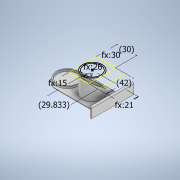
# Autodesk Inventor part: RV
Saved by Autodesk Inventor 2021 (Build 250183000, 183)
## iProperties
Created: 2020-06-05
Part Number: RV
Material: Generic
Document SubType Name: Modeling
Designer: andre
Density: 1 g/cm^3
Appearance: Default
Author: andre
## iProperties of the stored document _3DPrint.ipt
Created: 2020-06-05
Part Number: _3DPrint
Material: Generic
Document SubType Name: Modeling
Designer: andre
Density: 1 g/cm^3
Appearance: Default
Author: andre
Autodesk Inventor part; units mm, degrees
ref_plane "YZ Plane" through (0, 0, 0) normal (1, 0, 0) x (0, 1, 0)
ref_plane "XZ Plane" through (0, 0, 0) normal (0, 1, 0) x (-1, 0, 0)
ref_plane "XY Plane" through (0, 0, 0) normal (0, 0, 1) x (1, 0, 0)
sketch "Sketch1" plane through (0, 0, 0) normal (0, 1, 0) x (-1, 0, 0)
  line L0 (0, 0) -> (85, 0)
  line L1 (85, 0) -> (85, -42)
  line L2 (85, -42) -> (0, -42)
  line L3 (0, -42) -> (0, 0)
  dimension "d0" = 85
  dimension "d1" = 42
  constraints: 8 end point, 2 parallel, 1 horizontal, 1 perpendicular
  measures "d0" distance of L1.end L2.end
  measures "d1" distance of L0.end L1.end
extrude "Extrusion1" add sketch "Sketch1" along normal blind 1
sketch "Sketch2" plane through (0, 1, 0) normal (0, 1, 0) x (1, 0, 0)
  line L0 (-44.8327, 0) -> (-14.8327, 0)
  line L1 (-14.8327, 0) -> (-14.8327, 42)
  line L2 (-14.8327, 42) -> (-44.8327, 42)
  line L3 (-44.8327, 42) -> (-44.8327, 0)
  line L4 (-85, 0) -> (0, 0) projected
  dimension "d4" = 42
  dimension "d5" = 30
  dimension "d6" = 0
  constraints: 8 end point, 2 parallel, 1 horizontal, 1 perpendicular
  measures "d4" distance between parallel lines of L2 L0
  measures "d5" distance between parallel lines of L1 L3
  measures "d6" distance between parallel lines of L4 L0
extrude "Extrusion2" add sketch "Sketch2" along normal blind 32
sketch "Sketch5" plane through (0, 33, 0) normal (0, 1, 0) x (1, 0, 0)
  circle A0 centre (-29.8327, 21) radius 13
  line L0 (-44.8327, 42) -> (-44.8327, 0) projected
  line L1 (-44.8327, 0) -> (-14.8327, 0) projected
  line L2 (-14.8327, 0) -> (-14.8327, 42) projected
  line L3 (-14.8327, 42) -> (-44.8327, 42) projected
  circle A1 centre (-29.8327, 21) radius 15
  line L4 (0, 0) -> (0, 42) projected
  point P0 (-24.115, 0)
  point P1 (-44.8327, 21)
  point P2 (-14.8327, 21)
  point P3 (-19.6709, 0)
  dimension "d20" = 26
  dimension "d21" = 15
  dimension "d22" = 21
  dimension "d23" = 30
  dimension "d24" = 42
  dimension "d34" = 30
  dimension "d63" = 29.8327
  constraints: 2 centre point, 1 coincident
  measures "d20" diameter of A0
  measures "d21" distance from line of L0 A0.centre
  measures "d22" distance from line of L1 A0.centre
  measures "d23" distance between parallel lines of L2 L0
  measures "d24" distance between parallel lines of L3 L1
  measures "d34" diameter of A1
  measures "d63" distance from line of L4 A0.centre
extrude "Extrusion3" cut sketch "Sketch5" against normal blind 32 contours A0
chamfer "Chamfer3" distance 42 distance2 32 1 edges at (-29.8327, 33, -42)
extrude "Extrusion4" cut sketch "Sketch5" against normal blind 32 contours L3 L2 A1 L0 | A1 L2 L1 L0
sketch "Sketch6" plane through (0, 1, 0) normal (0, 1, 0) x (1, 0, 0)
  circle A0 centre (-68, 21) radius 15.75
  line L0 (-85, 0) -> (0, 0) projected
  circle A1 centre (-68, 21) radius 17
  line L1 (-85, 42) -> (-85, 0) projected
  point P0 (-28.5591, 0)
  dimension "d37" = 31.5
  dimension "d38" = 21
  dimension "d39" = 34
  dimension "d64" = 17
  constraints: 2 centre point, 1 coincident
  measures "d37" diameter of A0
  measures "d38" distance from line of L0 A0.centre
  measures "d39" diameter of A1
  measures "d64" distance from line of L1 A1.centre
extrude "Extrusion5" add sketch "Sketch6" along normal blind 3
fillet "Fillet3" radius 21 2 edges at (-85, 0.5, 0) (-85, 0.5, -42)
sketch "Sketch9" plane through (0, 0, 0) normal (1, 0, 0) x (0, 0, -1)
  line L0 (-11.5, 0) -> (53.5, 0)
  line L1 (53.5, 0) -> (53.5, 1)
  line L2 (53.5, 1) -> (-11.5, 1)
  line L3 (-11.5, 1) -> (-11.5, 0)
  line L4 (0, 0) -> (0, 1) projected
  dimension "d49" = 1
  dimension "d50" = 65
  dimension "d53" = 11.5
  constraints: 8 end point, 2 parallel, 1 horizontal, 1 perpendicular
  measures "d49" distance of L1.end L0.end
  measures "d50" distance between parallel lines of L1 L3
  measures "d53" distance between parallel lines of L3 L4
extrude "Extrusion8" add sketch "Sketch9" along normal blind 2
sketch "Sketch10" plane through (0, 1, 0) normal (0, 1, 0) x (1, 0, 0)
  line L0 (0, -11.5) -> (0, 0) projected
  line L1 (2, 53.5) -> (2, -11.5) projected
  line L2 (0, -11.5) -> (2, -11.5)
  line L3 (2, -11.5) -> (2, 53.5)
  line L4 (2, 53.5) -> (0, 53.5)
  line L5 (0, 53.5) -> (0, -11.5)
  point P0 (2, -11.5)
  constraints: 8 end point, 2 parallel, 1 horizontal, 1 perpendicular
extrude "Extrusion9" add sketch "Sketch10" along normal blind 15
sketch "Sketch11" plane through (0, 0, 0) normal (-1, 0, 0) x (0, 0, 1)
  line L0 (11.5, 0) -> (-53.5, 0) projected
  line L1 (-53.5, 6) -> (-42, 6)
  line L2 (-42, 6) -> (-42, 0)
  line L3 (-42, 0) -> (-53.5, 0)
  line L4 (-53.5, 0) -> (-53.5, 6)
  line L5 (-53.5, 16) -> (11.5, 16) projected
  line L6 (-53.5, 0) -> (-53.5, 16) projected
  point P0 (0, 0)
  dimension "d56" = 11.5
  dimension "d58" = 0
  dimension "d65" = 6
  constraints: 8 end point, 2 parallel, 1 horizontal, 1 perpendicular, 1 point on line
  measures "d56" distance of L2.end L3.end
  measures "d58" distance between parallel lines of L6 L4
  measures "d65" distance between parallel lines of L1 L0
extrude "Extrusion10" add sketch "Sketch11" along normal blind 6
fillet "Fillet4" radius 5.9 1 edges at (-6, 6, -47.75)
fillet "Fillet5" radius 2 1 edges at (2, 16, -21)
sketch "Sketch12" plane through (0, 1, 0) normal (0, 1, 0) x (1, 0, 0)
  line L0 (-4.5, 34) -> (-10.3327, 34)
  line L1 (-10.3327, 34) -> (-10.3327, 8)
  line L2 (-10.3327, 8) -> (-4.5, 8)
  line L3 (-4.5, 8) -> (-4.5, 34)
  line L4 (-5.931, 42) -> (-64, 42) projected
  line L5 (-64, 0) -> (0, 0) projected
  line L6 (0, 53.5) -> (0, -11.5) projected
  circle A0 centre (-29.8327, 21) radius 15 projected
  dimension "d66" = 8
  dimension "d67" = 8
  dimension "d68" = 4.5
  dimension "d69" = 4.5
  constraints: 8 end point, 2 parallel, 1 horizontal, 1 perpendicular
  measures "d66" distance between parallel lines of L4 L0
  measures "d67" distance between parallel lines of L5 L2
  measures "d68" distance between parallel lines of L6 L3
  measures "d69" distance edge to line of A0 L1
extrude "Extrusion11" add sketch "Sketch12" along normal blind 2 contours L3 L2 L1 L0
sketch "Sketch13" plane through (0, 3, 0) normal (0, 1, 0) x (1, 0, 0)
  line L0 (-4.5, 34) -> (-4.5, 8) construction
  line L1 (-4.5, 8) -> (-10.3327, 8) construction
  line L2 (-10.3327, 8) -> (-10.3327, 34) construction
  line L3 (-10.3327, 34) -> (-4.5, 34) construction
  line L4 (-4.5, 34) -> (-10.3327, 34) projected
  line L5 (-10.3327, 8) -> (-4.5, 8) projected
  line L6 (-4.5, 8) -> (-4.5, 34) projected
  line L7 (-10.3327, 34) -> (-10.3327, 8) projected
  spline S0 degree 2 poles (-8.9212, 32.0386) (-8.9188, 31.8937) (-8.7545, 31.7343) (-8.6024, 31.7319) knots 0 0 0 1 2 2 2
  line L8 (-8.6024, 31.7319) -> (-7.8101, 31.7319)
  line L9 (-7.8101, 31.7319) -> (-7.8101, 31.2126)
  line L10 (-7.8101, 31.2126) -> (-8.6893, 30.7271)
  spline S1 degree 2 poles (-8.6893, 30.7271) (-8.8197, 30.657) (-8.9236, 30.5217) (-8.9212, 30.4155) knots 0 0 0 1 2 2 2
  spline S2 degree 2 poles (-8.9212, 30.4155) (-8.9188, 30.2802) (-8.7642, 30.1111) (-8.641, 30.1063) knots 0 0 0 1 2 2 2
  spline S3 degree 2 poles (-8.641, 30.1063) (-8.5903, 30.1063) (-8.4937, 30.1353) (-8.4309, 30.1715) knots 0 0 0 1 2 2 2
  line L11 (-8.4309, 30.1715) -> (-7.7014, 30.5942)
  spline S4 degree 2 poles (-7.7014, 30.5942) (-7.5951, 30.3502) (-7.1652, 30.0918) (-6.8874, 30.0918) knots 0 0 0 1 2 2 2
  spline S5 degree 2 poles (-6.8874, 30.0918) (-6.4502, 30.0942) (-5.9623, 30.6401) (-5.9574, 31.1473) knots 0 0 0 1 2 2 2
  line L12 (-5.9574, 31.1473) -> (-5.9574, 32.0386)
  spline S6 degree 2 poles (-5.9574, 32.0386) (-5.9574, 32.1836) (-6.1241, 32.343) (-6.2738, 32.343) knots 0 0 0 1 2 2 2
  line L13 (-6.2738, 32.343) -> (-8.6024, 32.343)
  spline S7 degree 2 poles (-8.6024, 32.343) (-8.7545, 32.343) (-8.9188, 32.1836) (-8.9212, 32.0386) knots 0 0 0 1 2 2 2
  line L14 (-7.3656, 31.7319) -> (-6.4357, 31.7319)
  line L15 (-6.4357, 31.7319) -> (-6.4357, 31.2126)
  spline S8 degree 2 poles (-6.4357, 31.2126) (-6.4381, 30.9831) (-6.6845, 30.7222) (-6.8995, 30.7198) knots 0 0 0 1 2 2 2
  spline S9 degree 2 poles (-6.8995, 30.7198) (-7.1193, 30.7198) (-7.3632, 30.9734) (-7.3656, 31.2077) knots 0 0 0 1 2 2 2
  line L16 (-7.3656, 31.2077) -> (-7.3656, 31.7319)
  spline S10 degree 2 poles (-8.9164, 29.4179) (-8.9164, 29.2899) (-8.7666, 29.1473) (-8.6313, 29.1473) knots 0 0 0 1 2 2 2
  line L17 (-8.6313, 29.1473) -> (-6.9067, 29.1473)
  line L18 (-6.9067, 29.1473) -> (-6.9067, 29.1304)
  line L19 (-6.9067, 29.1304) -> (-8.6748, 28.4082)
  spline S11 degree 2 poles (-8.6748, 28.4082) (-8.769, 28.372) (-8.8608, 28.2391) (-8.8584, 28.1425) knots 0 0 0 1 2 2 2
  spline S12 degree 2 poles (-8.8584, 28.1425) (-8.8608, 28.0483) (-8.769, 27.9203) (-8.6724, 27.8816) knots 0 0 0 1 2 2 2
  line L20 (-8.6724, 27.8816) -> (-6.9067, 27.1594)
  line L21 (-6.9067, 27.1594) -> (-6.9067, 27.1425)
  line L22 (-6.9067, 27.1425) -> (-8.6313, 27.1425)
  spline S13 degree 2 poles (-8.6313, 27.1425) (-8.7666, 27.1425) (-8.9164, 27.0024) (-8.9164, 26.872) knots 0 0 0 1 2 2 2
  spline S14 degree 2 poles (-8.9164, 26.872) (-8.9164, 26.7415) (-8.7666, 26.599) (-8.6313, 26.599) knots 0 0 0 1 2 2 2
  line L23 (-8.6313, 26.599) -> (-6.3101, 26.599)
  spline S15 degree 2 poles (-6.3101, 26.599) (-6.1241, 26.6014) (-5.9188, 26.8043) (-5.9164, 26.9928) knots 0 0 0 1 2 2 2
  spline S16 degree 2 poles (-5.9164, 26.9928) (-5.9164, 27.1498) (-6.0661, 27.3502) (-6.2328, 27.4155) knots 0 0 0 1 2 2 2
  line L24 (-6.2328, 27.4155) -> (-8.0275, 28.1377)
  line L25 (-8.0275, 28.1377) -> (-8.0275, 28.1546)
  line L26 (-8.0275, 28.1546) -> (-6.2328, 28.8792)
  spline S17 degree 2 poles (-6.2328, 28.8792) (-6.0637, 28.942) (-5.9139, 29.1401) (-5.9164, 29.2971) knots 0 0 0 1 2 2 2
  spline S18 degree 2 poles (-5.9164, 29.2971) (-5.9188, 29.4855) (-6.1241, 29.6908) (-6.3101, 29.6908) knots 0 0 0 1 2 2 2
  line L27 (-6.3101, 29.6908) -> (-8.6313, 29.6908)
  spline S19 degree 2 poles (-8.6313, 29.6908) (-8.7666, 29.6908) (-8.9164, 29.5483) (-8.9164, 29.4179) knots 0 0 0 1 2 2 2
  line L28 (-8.8777, 24.9903) -> (-8.8777, 24.0024)
  spline S20 degree 2 poles (-8.8777, 24.0024) (-8.8729, 23.529) (-8.4309, 22.9976) (-8.042, 22.9928) knots 0 0 0 1 2 2 2
  spline S21 degree 2 poles (-8.042, 22.9928) (-7.7473, 22.9976) (-7.3632, 23.3768) (-7.3342, 23.6812) knots 0 0 0 1 2 2 2
  line L29 (-7.3342, 23.6812) -> (-7.3197, 23.6812)
  spline S22 degree 2 poles (-7.3197, 23.6812) (-7.2787, 23.442) (-6.9309, 23.1377) (-6.6845, 23.1329) knots 0 0 0 1 2 2 2
  spline S23 degree 2 poles (-6.6845, 23.1329) (-6.3463, 23.1353) (-5.9598, 23.6087) (-5.9574, 24.0242) knots 0 0 0 1 2 2 2
  line L30 (-5.9574, 24.0242) -> (-5.9574, 24.9903)
  spline S24 degree 2 poles (-5.9574, 24.9903) (-5.9574, 25.1353) (-6.1241, 25.2947) (-6.2738, 25.2947) knots 0 0 0 1 2 2 2
  line L31 (-6.2738, 25.2947) -> (-8.5589, 25.2947)
  spline S25 degree 2 poles (-8.5589, 25.2947) (-8.711, 25.2947) (-8.8777, 25.1353) (-8.8777, 24.9903) knots 0 0 0 1 2 2 2
  line L32 (-8.4212, 24.6836) -> (-7.5734, 24.6836)
  line L33 (-7.5734, 24.6836) -> (-7.5734, 24.1715)
  spline S26 degree 2 poles (-7.5734, 24.1715) (-7.5758, 23.901) (-7.7883, 23.6159) (-7.9937, 23.6159) knots 0 0 0 1 2 2 2
  spline S27 degree 2 poles (-7.9937, 23.6159) (-8.2038, 23.6159) (-8.4212, 23.8937) (-8.4212, 24.1594) knots 0 0 0 1 2 2 2
  line L34 (-8.4212, 24.1594) -> (-8.4212, 24.6836)
  line L35 (-7.1724, 24.6836) -> (-6.4115, 24.6836)
  line L36 (-6.4115, 24.6836) -> (-6.4115, 24.1836)
  spline S28 degree 2 poles (-6.4115, 24.1836) (-6.4139, 23.9662) (-6.6048, 23.7343) (-6.7811, 23.7343) knots 0 0 0 1 2 2 2
  spline S29 degree 2 poles (-6.7811, 23.7343) (-6.9671, 23.7343) (-7.17, 24) (-7.1724, 24.2464) knots 0 0 0 1 2 2 2
  line L37 (-7.1724, 24.2464) -> (-7.1724, 24.6836)
  spline S30 degree 2 poles (-8.9164, 22.4493) (-8.9164, 22.3285) (-8.7859, 22.1812) (-8.641, 22.1401) knots 0 0 0 1 2 2 2
  line L38 (-8.641, 22.1401) -> (-8.1845, 21.9855)
  line L39 (-8.1845, 21.9855) -> (-8.1845, 20.9324)
  line L40 (-8.1845, 20.9324) -> (-8.6458, 20.7778)
  spline S31 degree 2 poles (-8.6458, 20.7778) (-8.7883, 20.7367) (-8.9164, 20.587) (-8.9164, 20.4589) knots 0 0 0 1 2 2 2
  spline S32 degree 2 poles (-8.9164, 20.4589) (-8.9139, 20.3237) (-8.7569, 20.157) (-8.6289, 20.1546) knots 0 0 0 1 2 2 2
  spline S33 degree 2 poles (-8.6289, 20.1546) (-8.583, 20.1546) (-8.4937, 20.1715) (-8.4333, 20.1932) knots 0 0 0 1 2 2 2
  line L41 (-8.4333, 20.1932) -> (-6.2618, 20.9952)
  spline S34 degree 2 poles (-6.2618, 20.9952) (-6.083, 21.058) (-5.9164, 21.2826) (-5.9164, 21.4614) knots 0 0 0 1 2 2 2
  spline S35 degree 2 poles (-5.9164, 21.4614) (-5.9164, 21.6329) (-6.0854, 21.8575) (-6.2618, 21.9203) knots 0 0 0 1 2 2 2
  line L42 (-6.2618, 21.9203) -> (-8.4333, 22.7174)
  spline S36 degree 2 poles (-8.4333, 22.7174) (-8.4912, 22.7391) (-8.5903, 22.7585) (-8.6289, 22.7585) knots 0 0 0 1 2 2 2
  spline S37 degree 2 poles (-8.6289, 22.7585) (-8.7618, 22.7585) (-8.9139, 22.5942) (-8.9164, 22.4493) knots 0 0 0 1 2 2 2
  line L43 (-7.711, 21.8527) -> (-6.5154, 21.4734)
  line L44 (-6.5154, 21.4734) -> (-6.5154, 21.4589)
  line L45 (-6.5154, 21.4589) -> (-7.711, 21.0725)
  line L46 (-7.711, 21.0725) -> (-7.711, 21.8527)
  spline S38 degree 2 poles (-8.926, 18.715) (-8.9212, 18.1643) (-8.4284, 17.5435) (-7.9961, 17.5386) knots 0 0 0 1 2 2 2
  spline S39 degree 2 poles (-7.9961, 17.5386) (-7.6652, 17.5362) (-7.269, 17.9638) (-7.1796, 18.4251) knots 0 0 0 1 2 2 2
  line L47 (-7.1796, 18.4251) -> (-7.1168, 18.7343)
  spline S40 degree 2 poles (-7.1168, 18.7343) (-7.0661, 18.9903) (-6.8898, 19.2222) (-6.7569, 19.2198) knots 0 0 0 1 2 2 2
  spline S41 degree 2 poles (-6.7569, 19.2198) (-6.5927, 19.215) (-6.4019, 18.9469) (-6.3995, 18.7174) knots 0 0 0 1 2 2 2
  spline S42 degree 2 poles (-6.3995, 18.7174) (-6.3995, 18.529) (-6.5468, 18.2536) (-6.711, 18.1812) knots 0 0 0 1 2 2 2
  spline S43 degree 2 poles (-6.711, 18.1812) (-6.8052, 18.1304) (-6.8922, 17.9903) (-6.8922, 17.8889) knots 0 0 0 1 2 2 2
  spline S44 degree 2 poles (-6.8922, 17.8889) (-6.8898, 17.7705) (-6.7569, 17.6304) (-6.6482, 17.628) knots 0 0 0 1 2 2 2
  spline S45 degree 2 poles (-6.6482, 17.628) (-6.6072, 17.628) (-6.542, 17.6401) (-6.5106, 17.6498) knots 0 0 0 1 2 2 2
  spline S46 degree 2 poles (-6.5106, 17.6498) (-6.2231, 17.7512) (-5.9091, 18.3116) (-5.9067, 18.7174) knots 0 0 0 1 2 2 2
  spline S47 degree 2 poles (-5.9067, 18.7174) (-5.9091, 19.0435) (-6.1289, 19.5459) (-6.5251, 19.8285) (-6.7956, 19.8333) knots 0 0 0 1 2 3 3 3
  spline S48 degree 2 poles (-6.7956, 19.8333) (-7.1217, 19.8333) (-7.5371, 19.401) (-7.6241, 18.9638) knots 0 0 0 1 2 2 2
  line L48 (-7.6241, 18.9638) -> (-7.6845, 18.6546)
  spline S49 degree 2 poles (-7.6845, 18.6546) (-7.74, 18.3816) (-7.9188, 18.1473) (-8.0613, 18.1498) knots 0 0 0 1 2 2 2
  spline S50 degree 2 poles (-8.0613, 18.1498) (-8.2255, 18.1546) (-8.4309, 18.4517) (-8.4333, 18.7005) knots 0 0 0 1 2 2 2
  spline S51 degree 2 poles (-8.4333, 18.7005) (-8.4357, 18.913) (-8.2763, 19.2295) (-8.1096, 19.3043) knots 0 0 0 1 2 2 2
  spline S52 degree 2 poles (-8.1096, 19.3043) (-8.0154, 19.3575) (-7.9309, 19.4928) (-7.9333, 19.5845) knots 0 0 0 1 2 2 2
  spline S53 degree 2 poles (-7.9333, 19.5845) (-7.9333, 19.7053) (-8.0782, 19.8527) (-8.2014, 19.8551) knots 0 0 0 1 2 2 2
  spline S54 degree 2 poles (-8.2014, 19.8551) (-8.2424, 19.8551) (-8.327, 19.8382) (-8.3656, 19.8213) knots 0 0 0 1 2 2 2
  spline S55 degree 2 poles (-8.3656, 19.8213) (-8.6096, 19.7319) (-8.9212, 19.1691) (-8.926, 18.715) knots 0 0 0 1 2 2 2
  line L49 (-8.8777, 16.8623) -> (-8.8777, 15.4734)
  spline S56 degree 2 poles (-8.8777, 15.4734) (-8.8777, 15.3454) (-8.7449, 15.1981) (-8.6241, 15.1957) knots 0 0 0 1 2 2 2
  spline S57 degree 2 poles (-8.6241, 15.1957) (-8.5057, 15.1981) (-8.3729, 15.3478) (-8.3729, 15.4734) knots 0 0 0 1 2 2 2
  line L50 (-8.3729, 15.4734) -> (-8.3729, 16.5556)
  line L51 (-8.3729, 16.5556) -> (-7.6338, 16.5556)
  line L52 (-7.6338, 16.5556) -> (-7.6338, 15.5266)
  spline S58 degree 2 poles (-7.6338, 15.5266) (-7.6338, 15.4082) (-7.5106, 15.2729) (-7.3995, 15.2705) knots 0 0 0 1 2 2 2
  spline S59 degree 2 poles (-7.3995, 15.2705) (-7.2908, 15.2729) (-7.1652, 15.4106) (-7.1652, 15.5266) knots 0 0 0 1 2 2 2
  line L53 (-7.1652, 15.5266) -> (-7.1652, 16.5556)
  line L54 (-7.1652, 16.5556) -> (-6.4623, 16.5556)
  line L55 (-6.4623, 16.5556) -> (-6.4623, 15.4734)
  spline S60 degree 2 poles (-6.4623, 15.4734) (-6.4623, 15.3478) (-6.3294, 15.1981) (-6.211, 15.1957) knots 0 0 0 1 2 2 2
  spline S61 degree 2 poles (-6.211, 15.1957) (-6.0903, 15.1981) (-5.9574, 15.3454) (-5.9574, 15.4734) knots 0 0 0 1 2 2 2
  line L56 (-5.9574, 15.4734) -> (-5.9574, 16.8623)
  spline S62 degree 2 poles (-5.9574, 16.8623) (-5.9574, 17.0072) (-6.1241, 17.1667) (-6.2738, 17.1667) knots 0 0 0 1 2 2 2
  line L57 (-6.2738, 17.1667) -> (-8.5589, 17.1667)
  spline S63 degree 2 poles (-8.5589, 17.1667) (-8.711, 17.1667) (-8.8777, 17.0072) (-8.8777, 16.8623) knots 0 0 0 1 2 2 2
  spline S64 degree 2 poles (-8.9164, 12.8092) (-8.9164, 12.6328) (-8.7473, 12.4082) (-8.5637, 12.343) knots 0 0 0 1 2 2 2
  line L58 (-8.5637, 12.343) -> (-6.3608, 11.5242)
  spline S65 degree 2 poles (-6.3608, 11.5242) (-6.2787, 11.4952) (-6.199, 11.4952) knots 0 0 0 1 1 1
  spline S66 degree 2 poles (-6.199, 11.4952) (-6.0709, 11.4976) (-5.9188, 11.6667) (-5.9164, 11.8092) knots 0 0 0 1 2 2 2
  spline S67 degree 2 poles (-5.9164, 11.8092) (-5.9164, 11.9275) (-6.0299, 12.0725) (-6.1507, 12.1111) knots 0 0 0 1 2 2 2
  line L59 (-6.1507, 12.1111) -> (-8.2473, 12.7923)
  line L60 (-8.2473, 12.7923) -> (-8.2473, 12.8068)
  line L61 (-8.2473, 12.8068) -> (-6.1579, 13.4903)
  spline S68 degree 2 poles (-6.1579, 13.4903) (-6.0323, 13.5266) (-5.9164, 13.6787) (-5.9164, 13.8019) knots 0 0 0 1 2 2 2
  spline S69 degree 2 poles (-5.9164, 13.8019) (-5.9188, 13.9493) (-6.0758, 14.1208) (-6.2062, 14.1232) knots 0 0 0 1 2 2 2
  spline S70 degree 2 poles (-6.2062, 14.1232) (-6.2932, 14.1232) (-6.3777, 14.0942) knots 0 0 0 1 1 1
  line L62 (-6.3777, 14.0942) -> (-8.5613, 13.2802)
  spline S71 degree 2 poles (-8.5613, 13.2802) (-8.7473, 13.215) (-8.9164, 12.9879) (-8.9164, 12.8092) knots 0 0 0 1 2 2 2
  spline S72 degree 2 poles (-8.9212, 10.1643) (-8.9188, 10.0266) (-8.7545, 9.8647) (-8.6144, 9.8623) knots 0 0 0 1 2 2 2
  line L63 (-8.6144, 9.8623) -> (-6.2545, 9.8623)
  spline S73 degree 2 poles (-6.2545, 9.8623) (-6.0951, 9.8647) (-5.9139, 10.0459) (-5.9115, 10.2101) knots 0 0 0 1 2 2 2
  spline S74 degree 2 poles (-5.9115, 10.2101) (-5.9115, 10.3019) (-5.9574, 10.4686) (-6.0275, 10.5725) knots 0 0 0 1 2 2 2
  line L64 (-6.0275, 10.5725) -> (-6.4284, 11.1522)
  spline S75 degree 2 poles (-6.4284, 11.1522) (-6.4792, 11.2222) (-6.5879, 11.285) (-6.6579, 11.285) knots 0 0 0 1 2 2 2
  spline S76 degree 2 poles (-6.6579, 11.285) (-6.7569, 11.2826) (-6.8753, 11.1643) (-6.8753, 11.07) knots 0 0 0 1 2 2 2
  spline S77 degree 2 poles (-6.8753, 11.07) (-6.8753, 11.0242) (-6.8511, 10.9493) (-6.8222, 10.9082) knots 0 0 0 1 2 2 2
  line L65 (-6.8222, 10.9082) -> (-6.5226, 10.4807)
  line L66 (-6.5226, 10.4807) -> (-6.5226, 10.4686)
  line L67 (-6.5226, 10.4686) -> (-8.6144, 10.4686)
  spline S78 degree 2 poles (-8.6144, 10.4686) (-8.7545, 10.4662) (-8.9188, 10.3019) (-8.9212, 10.1643) knots 0 0 0 1 2 2 2
  point P0 (0, 0)
  dimension "d72" = 0
  dimension "d73" = 0
  dimension "d74" = 0
  dimension "d75" = 0
  constraints: 2 other
  measures "d72" distance between parallel lines of L4 L3
  measures "d73" distance between parallel lines of L5 L1
  measures "d74" distance between parallel lines of L6 L0
  measures "d75" distance between parallel lines of L7 L2
extrude "Extrusion12" cut sketch "Sketch13" against normal blind 2 contours S7 L13 S6 L12 S5 S4 L11 S3 S2 S1 L10 L9 L8 S0 | S19 L27 S18 S17 L26 L25 L24 S16 S15 L23 S14 S13 L22 L21 L20 S12 S11 L19 L18 L17 S10 | S25 L31 S24 L30 S23 S22 L29 S21 S20 L28 | S37 S36 L42 S35 S34 L41 S33 S32 S31 L40 L39 L38 S30 | S55 S54 S53 S52 S51 S50 S49 L48 S48 S47 S46 S45 S44 S43 S42 S41 S40 L47 S39 S38 | S63 L57 S62 L56 S61 S60 L55 L54 L53 S59 S58 L52 L51 L50 S57 S56 L49 | S71 L62 S70 S69 S68 L61 L60 L59 S67 S66 S65 L58 S64 | S78 L67 L66 L65 S77 S76 S75 L64 S74 S73 L63 S72
equation "\"d4\" = d1"
equation "\"d21\" = 0.5 * d23"
equation "\"d22\" = 0.5 * d1"
equation "\"d34\" = d23"
equation "\"d25\" = d7"
equation "\"d30\" = d1"
equation "\"d31\" = d7"
equation "\"d38\" = 0.5 * d1"
equation "\"d64\" = 0.5 * d39"
equation "\"d42\" = 0.5 * d1"
equation "\"d53\" = -0.5 * d1 + 0.5 * d50"
equation "\"d56\" = d53"
equation "\"d67\" = d66"
equation "\"d69\" = d68"
equation "\"d7\" = 32"
body "Solid1"
